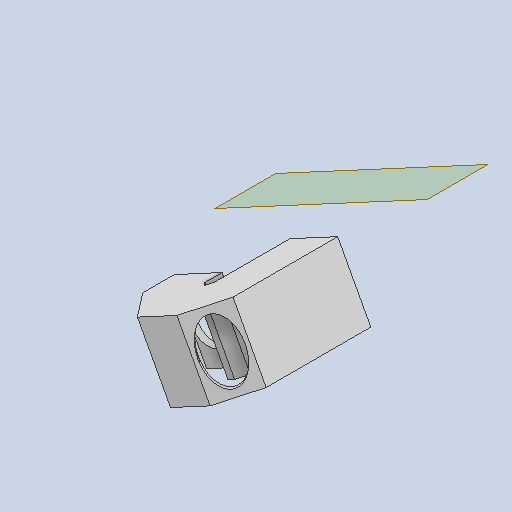
# Autodesk Inventor part: Matchboxscope_Lightperiscope_V0
Saved by Autodesk Inventor 2022 (Build 260153000, 153)
## iProperties
Created: 2022-03-26
Part Number: Matchboxscope_Lightperiscope_V0
Material: Generic
Document SubType Name: Modeling
Designer: Prakash Lab
Density: 1 g/cm^3
Appearance: Default
Author: Prakash Lab
Autodesk Inventor part; units mm, degrees
ref_plane "YZ Plane" through (0, 0, 0) normal (1, 0, 0) x (0, 1, 0)
ref_plane "XZ Plane" through (0, 0, 0) normal (0, 1, 0) x (-1, 0, 0)
ref_plane "XY Plane" through (0, 0, 0) normal (0, 0, 1) x (1, 0, 0)
ref_plane "Work Plane1" through (118.9518, 9.9874, -13.1749) normal (0.4728584, -0.8811384, 0) x (0, 0, -1)
sketch "Sketch1" plane through (118.9518, 9.9874, -13.1749) normal (0.4728584, -0.8811384, 0) x (0, 0, -1)
  line L0 (-0.7641, 6) -> (-0.7641, -6)
  line L1 (-16.5984, 5.4988) -> (-16.5984, 6)
  line L2 (-7.5984, -7.7203) -> (-5.5984, -7.7203)
  line L3 (-7.5984, -21.1989) -> (-0.5984, -21.1989)
  line L4 (-1.2281, -14.4596) -> (-31.7652, -14.4596) construction
  line L5 (-16.5984, 11.5008) -> (-16.5984, -0.9971) projected
  line L6 (-15.5984, -2) -> (-12.5984, -2)
  line L7 (-16.5984, 2) -> (-12.5984, 2)
  line L8 (-16.5984, -5.9845) -> (-33.3752, -5.9845)
  line L9 (-33.3752, -5.9845) -> (-34.3463, -6.9556)
  line L10 (-34.3463, -6.9556) -> (-34.3463, -7.3626)
  line L11 (-34.3463, -7.3626) -> (-33.2494, -8.4596)
  line L12 (-33.2494, -8.4596) -> (-29.4011, -8.4596)
  line L13 (-29.4011, -8.4596) -> (-29.4011, -20.4596)
  line L14 (-29.4011, -20.4596) -> (-36.385, -20.4596)
  line L15 (-36.385, -20.4596) -> (-46.3463, -10.4983)
  line L16 (-46.3463, -10.4983) -> (-46.3463, -0.5819)
  line L17 (-46.3463, -0.5819) -> (-39.7488, 6.0155)
  line L18 (-39.7488, 6.0155) -> (-16.5984, 6.0155)
  line L19 (-16.5984, -5.9845) -> (-16.5984, 6.0155)
  line L20 (-16.5984, 0.0155) -> (-32.985, 0.0155) construction
  point P0 (-13.1749, -109.5356)
  dimension "d22" = 13.4786
  dimension "d23" = 6.7393
  dimension "d24" = 135
  dimension "d25" = 135
  dimension "d26" = 4
  dimension "d27" = 6
  dimension "d28" = 6
  dimension "d29" = 6
  dimension "d30" = 6
  dimension "d31" = 12
  constraints: 40 end point, 7 horizontal, 6 perpendicular, 2 parallel, 1 collinear, 1 midpoint, 1 point on line, 10 other
  measures "d22" distance between parallel lines of L2 L3
  measures "d23" distance between parallel lines of L3 L4
  measures "d24" angle of L9 L8
  measures "d25" angle of L14 L15
  measures "d26" distance between parallel lines of L7 L6
  measures "d27" distance between parallel lines of L8 L20
  measures "d28" distance between parallel lines of L18 L20
  measures "d29" distance between parallel lines of L14 L4
  measures "d30" distance between parallel lines of L4 L12
  measures "d31" distance between parallel lines of L10 L16
extrude "Extrusion1" add sketch "Sketch1" along normal blind 1.5
sketch "Sketch2" plane through (119.6611, 8.6657, -13.1749) normal (0.4728584, -0.8811384, 0) x (0.8811384, 0.4728584, 0)
  line L0 (-0.5819, 46.3463) -> (-10.4983, 46.3463) projected
  line L1 (-10.4983, 46.3463) -> (-20.4596, 36.385) projected
  line L2 (-20.4596, 36.385) -> (-20.4596, 29.4011) projected
  line L3 (-20.4596, 29.4011) -> (-8.4596, 29.4011) projected
  line L4 (-8.4596, 29.4011) -> (-8.4596, 33.2494) projected
  line L5 (-8.4596, 33.2494) -> (-7.3626, 34.3463) projected
  line L6 (-7.3626, 34.3463) -> (-6.9556, 34.3463) projected
  line L7 (-6.9556, 34.3463) -> (-5.9845, 33.3752) projected
  line L8 (-5.9845, 33.3752) -> (-5.9845, 16.5984) projected
  line L9 (-5.9845, 16.5984) -> (6.0155, 16.5984) projected
  line L10 (6.0155, 16.5984) -> (6.0155, 39.7488) projected
  line L11 (6.0155, 39.7488) -> (-0.5819, 46.3463) projected
  line L12 (-18.9596, 35.7637) -> (-9.877, 44.8463)
  line L13 (-9.877, 44.8463) -> (-1.2032, 44.8463)
  line L14 (-1.2032, 44.8463) -> (4.5155, 39.1275)
  line L15 (4.5155, 39.1275) -> (4.5155, 18.0984)
  line L16 (4.5155, 18.0984) -> (-4.4845, 18.0984)
  line L17 (-4.4845, 18.0984) -> (-4.4845, 33.9965)
  line L18 (-4.4845, 33.9965) -> (-6.3342, 35.8463)
  line L19 (-6.3342, 35.8463) -> (-7.9839, 35.8463)
  line L20 (-7.9839, 35.8463) -> (-9.9596, 33.8707)
  line L21 (-9.9596, 33.8707) -> (-9.9596, 30.9011)
  line L22 (-9.9596, 30.9011) -> (-18.9596, 30.9011)
  line L23 (-18.9596, 30.9011) -> (-18.9596, 35.7637)
  point P0 (-109.5356, 13.1749)
  dimension "d32" = 1.5
  constraints: 24 end point, 11 other
  measures "d32" distance between parallel lines of L1 L12
extrude "Extrusion2" add sketch "Sketch2" along normal blind 14
sketch "Sketch3" plane through (103.7391, 1.8236, 16.2262) normal (0, 0, -1) x (-0.8811384, -0.4728584, 0)
  circle A0 centre (-2.8052, -7.75) radius 4.5
  line L0 (3.1948, 0) -> (-8.8052, 0) projected
  line L1 (-8.8052, 0) -> (-8.8052, -15.5) projected
  line L2 (3.1948, -15.5) -> (-8.8052, -15.5) projected
  line L3 (3.1948, 0) -> (3.1948, -15.5) projected
  point P0 (92.2708, 47.4471)
  constraints: 1 centre point
extrude "Extrusion3" cut sketch "Sketch3" against normal blind 1.5 contours A0
sketch "Sketch4" plane through (124.2386, 12.8245, 3.4235) normal (0, 0, 1) x (0.8811384, 0.4728584, 0)
  line L0 (-12, 0) -> (0, 0) projected
  line L1 (0, 0) -> (0, -15.5) projected
  line L2 (-12, 0) -> (-12, -15.5) projected
  circle A0 centre (-6, -7.75) radius 4.5
  line L3 (10.5, -15.5) -> (1.5, -15.5)
  line L4 (-12, -15.5) -> (0, -15.5) projected
  point P0 (-115.5356, 47.4471)
  constraints: 2 end point, 1 centre point, 1 horizontal
extrude "Extrusion4" cut sketch "Sketch4" along normal blind 1.5 contours A0
sketch "Sketch5" plane through (98.9794, -0.7307, 21.0031) normal (-0.623059, -0.3343614, 0.7071068) x (0.623059, 0.3343614, 0.7071068)
  line L0 (16.9706, 0) -> (0, 0) projected
  line L1 (0, 0) -> (0, -15.5) projected
  line L2 (16.9706, -15.5) -> (0, -15.5) projected
  line L3 (16.9706, 0) -> (16.9706, -15.5) projected
  ellipse E0 centre (9.9292, -7.5137) end of major axis (9.9292, -12.98) minor radius 6.3715
  line L4 (10.7303, 0) -> (10.7303, -15.5) projected
  point P0 (-76.2771, 47.4471)
  constraints: 1 centre point, 1 other
extrude "Extrusion5" cut sketch "Sketch5" against normal blind 1.5 contours L4 E0 | E0 L4
sketch "Sketch7" plane through (118.439, 9.7122, 33.1714) normal (0.623059, 0.3343614, 0.7071068) x (0.623059, 0.3343614, -0.7071068)
  line L0 (9.3302, 0) -> (9.3302, -15.5) projected
  line L1 (0, 0) -> (0, -15.5) projected
  line L2 (9.3302, 0) -> (0, 0) projected
  line L3 (9.3302, -15.5) -> (0, -15.5) projected
  ellipse E0 centre (4.6651, -7.75) end of major axis (4.6651, -1.4149) minor radius 3.942
  ellipse E1 centre (1.1084, -7.75) end of major axis (1.1084, -3.25) minor radius 3.182 (4.2904, -7.75) -> (-2.0735, -7.75) ccw projected
  point P0 (-53.5862, 47.4471)
  constraints: 3 other
extrude "Extrusion7" cut sketch "Sketch7" against normal blind 1.5 contours E0
equation "\"d23\" = 0.5 * d22"
body "Solid1"
